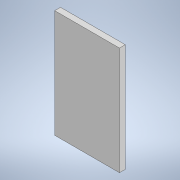
# Autodesk Inventor part: Maze part 5 (aurdino)
Saved by Autodesk Inventor 2021 (Build 250183000, 183)
## iProperties
Created: 2021-06-18
Part Number: Maze part 5 (aurdino)
Material: Generic
Document SubType Name: Modeling
Designer: Dell
Density: 1 g/cm^3
Appearance: Default
Author: Dell
Autodesk Inventor part; units mm, degrees
ref_plane "YZ Plane" through (0, 0, 0) normal (1, 0, 0) x (0, 1, 0)
ref_plane "XZ Plane" through (0, 0, 0) normal (0, 1, 0) x (-1, 0, 0)
ref_plane "XY Plane" through (0, 0, 0) normal (0, 0, 1) x (1, 0, 0)
sketch "Sketch1" plane through (0, 0, 0) normal (0, 0, 1) x (1, 0, 0)
  line L0 (-10.8775, 11.5546) -> (-6.4217, 11.5546)
  line L1 (-6.4217, 11.5546) -> (-6.4217, 4.1282)
  line L2 (-6.4217, 4.1282) -> (-10.8775, 4.1282)
  line L3 (-10.8775, 4.1282) -> (-10.8775, 11.5546)
  point P0 (0, 0)
  constraints: 8 end point, 2 parallel, 1 horizontal, 1 perpendicular
extrude "Extrusion1" add sketch "Sketch1" along normal blind 0.4
body "Solid1"
